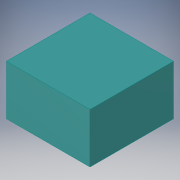
# Autodesk Inventor part: TPPAD1-13
Saved by Autodesk Inventor 2017.3 (Build 213256000, 256)
## iProperties
Part Number: TPPAD1-13
Material: Generisch
Document SubType Name: Modeling
Designer: Nils
Density: 1 g/cm^3
Appearance: P1-13, TPPAD1-13
Author: Nils
Autodesk Inventor part; units mm, degrees
ref_plane "YZ Plane" through (0, 0, 0) normal (1, 0, 0) x (0, 1, 0)
ref_plane "XZ Plane" through (0, 0, 0) normal (0, 1, 0) x (-1, 0, 0)
ref_plane "XY Plane" through (0, 0, 0) normal (0, 0, 1) x (1, 0, 0)
sketch "P1-13, TPPAD1-13_15" plane through (0, 0, 0) normal (0, 0, 1) x (1, 0, 0)
  line L0 (-0.8382, 0.8382) -> (0.8382, 0.8382)
  line L1 (0.8382, 0.8382) -> (0.8382, -0.8382)
  line L2 (0.8382, -0.8382) -> (-0.8382, -0.8382)
  line L3 (-0.8382, -0.8382) -> (-0.8382, 0.8382)
  constraints: 8 end point
extrude "Extrusion1" add sketch "P1-13, TPPAD1-13_15" along normal blind 1
